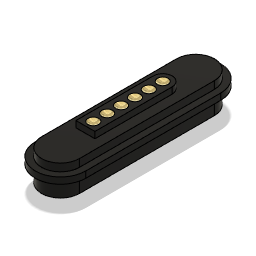
Printed glass bed Mod (Autodesk Fusion 360 archive; units mm, degrees)
design "6 pin megnegtic Pogo Pins"
Autodesk Fusion 360 part; units mm, degrees
sketch "Sketch1" plane through (0, 0, 0) normal (0, 1, 0) x (1, 0, 0)
  line L0 (-5.7502, 8.4443) -> (-5.7502, -12.9557)
  arc A0 (-5.7502, -12.9557) -> (2.2498, -12.9557) centre (-1.7502, -12.9557) ccw
  line L1 (2.2498, -12.9557) -> (2.2498, 8.4443)
  arc A1 (2.2498, 8.4443) -> (-5.7502, 8.4443) centre (-1.7502, 8.4443) ccw
  line L2 (-1.7502, 8.4443) -> (-1.7502, -12.9557) construction
  point P0 (-1.7502, 12.4443)
  point P1 (-1.7502, -16.9557)
  dimension "d1" = 29.4
  dimension "d2" = 8
  constraint tangent L0 A0
  constraint tangent A0 L1
  constraint parallel L0 L1
  constraint tangent L1 A1
  constraint tangent L0 A1
  constraint vertical L2
  constraint midpoint A1 P0
  constraint midpoint A0 P1
  measures "d1" distance of P0 P1
  measures "d2" distance of L0 L1
extrude "Extrude1" add sketch "Sketch1" along normal blind 1
sketch "Sketch2" plane through (0, 0, 0) normal (0, -1, 0) x (1, 0, 0)
  arc A0 (-5.7502, -8.4443) -> (2.2498, -8.4443) centre (-1.7502, -8.4443) ccw
  line L0 (2.2498, -8.4443) -> (2.2498, 12.9557)
  arc A1 (2.2498, 12.9557) -> (-5.7502, 12.9557) centre (-1.7502, 12.9557) ccw
  line L1 (-5.7502, 12.9557) -> (-5.7502, -8.4443)
  arc A2 (-4.7502, -8.4443) -> (1.2498, -8.4443) centre (-1.7502, -8.4443) ccw
  line L2 (1.2498, -8.4443) -> (1.2498, 12.9557)
  arc A3 (1.2498, 12.9557) -> (-4.7502, 12.9557) centre (-1.7502, 12.9557) ccw
  line L3 (-4.7502, 12.9557) -> (-4.7502, -8.4443)
  dimension "d5" = -1
  dimension "d6" = 6
  measures "d6" distance of L2 L3
extrude "Extrude2" add sketch "Sketch2" along normal blind 2.6 contours A2 L2 A3 L3
sketch "Sketch3" plane through (0, 1, 0) normal (0, 1, 0) x (-1, 0, 0)
  arc A0 (-2.2498, -8.4443) -> (5.7502, -8.4443) centre (1.7502, -8.4443) ccw
  line L0 (5.7502, -8.4443) -> (5.7502, 12.9557)
  arc A1 (5.7502, 12.9557) -> (-2.2498, 12.9557) centre (1.7502, 12.9557) ccw
  line L1 (-2.2498, 12.9557) -> (-2.2498, -8.4443)
  line L2 (1.7502, -12.4443) -> (1.7502, 16.9557) construction
  line L3 (0.2502, 7.7557) -> (0.2502, -3.2443)
  arc A2 (0.2502, -3.2443) -> (3.2502, -3.2443) centre (1.7502, -3.2443) ccw
  line L4 (3.2502, -3.2443) -> (3.2502, 7.7557)
  arc A3 (3.2502, 7.7557) -> (0.2502, 7.7557) centre (1.7502, 7.7557) ccw
  line L5 (1.7502, 7.7557) -> (1.7502, -3.2443) construction
  line L6 (3.2502, 7.7557) -> (3.2502, 9.0057)
  line L7 (3.2502, 9.0057) -> (0.2502, 9.0057)
  line L8 (0.2502, 9.0057) -> (0.2502, 7.7557)
  circle A4 centre (1.7502, -3.2443) radius 0.85
  circle A5 centre (1.7502, -1.0443) radius 0.85
  circle A6 centre (1.7502, 1.1557) radius 0.85
  circle A7 centre (1.7502, 3.3557) radius 0.85
  circle A8 centre (1.7502, 5.5557) radius 0.85
  circle A9 centre (1.7502, 7.7557) radius 0.85
  point P0 (1.7502, 2.2557)
  point P1 (1.7502, -4.7443)
  dimension "d9" = 7
  dimension "d10" = 3
  dimension "d11" = 1.25
  dimension "d12" = 5.5
  dimension "d13" = 1.7
  dimension "d16" = 0
  dimension "d17" = 11
  constraint midpoint A0 L2.start
  constraint midpoint A1 L2.end
  constraint tangent L3 A2
  constraint tangent A2 L4
  constraint parallel L3 L4
  constraint tangent L4 A3
  constraint tangent L3 A3
  constraint coincident L2 A2.centre
  constraint parallel L2 L5
  constraint midpoint L2 P0
  constraint midpoint L5 P0
  constraint midpoint A2 P1
  constraint tangent A3 L6
  constraint perpendicular L4 L7
  constraint vertical L8
  measures "d9" distance of P0 P1
  measures "d10" distance of L3 L4
  measures "d11" distance of A3.centre L7
  measures "d12" distance of P0 A2.centre
  measures "d13" diameter of A4
extrude "Extrude3" add sketch "Sketch3" along normal blind 2.2 contours L3 A2 L4 A3 L7 | A3 L7 L8 | A3 L6 L7 | A4 | A5 | A6 | A7 | A8 | A9
sketch "Sketch4" plane through (0, 1, 0) normal (0, 1, 0) x (-1, 0, 0)
  line L0 (0.2502, 9.0057) -> (3.2502, 9.0057)
  line L1 (3.2502, 9.0057) -> (3.2502, -3.2443)
  arc A0 (0.2502, -3.2443) -> (3.2502, -3.2443) centre (1.7502, -3.2443) ccw
  line L2 (0.2502, -3.2443) -> (0.2502, 9.0057)
  arc A1 (-2.2498, -8.4443) -> (5.7502, -8.4443) centre (1.7502, -8.4443) ccw
  line L3 (5.7502, -8.4443) -> (5.7502, 12.9557)
  arc A2 (5.7502, 12.9557) -> (-2.2498, 12.9557) centre (1.7502, 12.9557) ccw
  line L4 (-2.2498, 12.9557) -> (-2.2498, -8.4443)
  line L5 (4.7502, 12.9557) -> (4.7502, -8.4443)
  arc A3 (-1.2498, -8.4443) -> (4.7502, -8.4443) centre (1.7502, -8.4443) ccw
  line L6 (-1.2498, -8.4443) -> (-1.2498, 12.9557)
  arc A4 (4.7502, 12.9557) -> (-1.2498, 12.9557) centre (1.7502, 12.9557) ccw
extrude "Extrude4" add sketch "Sketch4" along normal blind 1.2 contours L5 A3 L6 A4
sketch "Sketch5" plane through (0, -2.6, 0) normal (0, -1, 0) x (1, 0, 0)
  line L0 (-4.7502, 12.9557) -> (-4.7502, -8.4443)
  arc A0 (-4.7502, -8.4443) -> (1.2498, -8.4443) centre (-1.7502, -8.4443) ccw
  line L1 (1.2498, -8.4443) -> (1.2498, 12.9557)
  arc A1 (1.2498, 12.9557) -> (-4.7502, 12.9557) centre (-1.7502, 12.9557) ccw
  line L2 (-0.2502, 9.0057) -> (-0.2502, -3.2443)
  arc A2 (-3.2502, -3.2443) -> (-0.2502, -3.2443) centre (-1.7502, -3.2443) ccw
  line L3 (-3.2502, -3.2443) -> (-3.2502, 9.0057)
  line L4 (-3.2502, 9.0057) -> (-0.2502, 9.0057)
  circle A3 centre (-1.7502, 7.7557) radius 0.5455
  circle A4 centre (-1.7502, 5.5557) radius 0.5
  circle A5 centre (-1.7502, 3.3557) radius 0.5
  circle A6 centre (-1.7502, 1.1557) radius 0.5
  circle A7 centre (-1.7502, -1.0443) radius 0.5
  circle A8 centre (-1.7502, -3.2443) radius 0.5
  dimension "d22" = 1
  constraint equal A7 A8
  constraint equal A6 A7
  constraint equal A5 A6
  constraint equal A4 A5
  measures "d22" diameter of A8
extrude "Extrude5" add sketch "Sketch5" along normal blind 1.5 contours A3 | A4 | A5 | A6 | A7 | A8
sketch "Sketch6" plane through (0, 3.2, 0) normal (0, 1, 0) x (-1, 0, 0)
  line L0 (0.2502, 9.0057) -> (0.2502, -3.2443)
  arc A0 (0.2502, -3.2443) -> (3.2502, -3.2443) centre (1.7502, -3.2443) ccw
  line L1 (3.2502, -3.2443) -> (3.2502, 9.0057)
  line L2 (3.2502, 9.0057) -> (0.2502, 9.0057)
  circle A1 centre (1.7502, 7.7557) radius 0.85
  line L3 (0.9002, 7.7557) -> (2.6002, 7.7557)
  point P0 (1.7502, 7.7557)
  constraint coincident A1 L3.start
  constraint coincident A1 L3.end
  constraint horizontal L3
  constraint coincident L3 P0
ref_plane "WorkPlane1" through (-1.7502, 3.2, 7.7557) normal (0, 0, 1) x (-1, 0, 0)
sketch "Sketch7" plane through (-1.7502, 3.2, 7.7557) normal (0, 0, 1) x (1, 0, 0)
  circle A0 centre (0, 1.2359) radius 1.5
  line L0 (1.5, 1.2359) -> (-1.5, 1.2359)
  point P0 (-0.85, 0)
  point P1 (0.85, 0)
  dimension "d26" = 3
  constraint coincident A0 P0
  constraint coincident A0 P1
  constraint coincident A0 L0.start
  constraint coincident A0 L0.end
  constraint horizontal L0
  constraint coincident A0.centre L0
  measures "d26" diameter of A0
revolve "Revolve1" cut sketch "Sketch7" angle 360 about axis through (-0.2502, 4.4359, 7.7557) along (-1, 0, 0) contours A0 L0 picked at (-0.3665, 0.8958)
pattern_linear "R-Pattern1" count 6 spacing 2.2 along (0, 0, -1) of "Revolve1"
